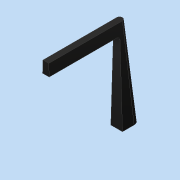
# Autodesk Inventor part: RudderStabilizingFins
Saved by Autodesk Inventor 2017 (Build 210142000, 142)
## iProperties
Created: 2016-10-10
Part Number: RudderStabilizingFins
Material: Generic
Document SubType Name: Modeling
Designer: techn
Density: 1 g/cm^3
Appearance: Glossy - Black
Author: techn
Autodesk Inventor part; units mm, degrees
ref_plane "YZ Plane" through (0, 0, 0) normal (1, 0, 0) x (0, 1, 0)
ref_plane "XY Plane" through (0, 0, 0) normal (0, 0, 1) x (1, 0, 0)
sketch "Sketch6" plane through (0, 0, 0) normal (0, 1, 0) x (-1, 0, 0)
  line L0 (0, 0) -> (6.35, 0)
  line L1 (6.35, 0) -> (6.35, -6.35)
  line L2 (6.35, -6.35) -> (0, -6.35)
  line L3 (0, -6.35) -> (0, 0)
  arc A0 (0, -6.35) -> (6.35, -6.35) centre (3.175, -6.35) ccw
  dimension "d25" = 6.35
  dimension "d26" = 6.35
  constraints: 8 end point, 2 parallel, 2 point on circle, 2 tangent, 1 centre point, 1 horizontal, 1 perpendicular
  measures "d25" distance of L1.end L2.end
  measures "d26" distance of L0.end L1.end
ref_plane "Work Plane1" through (0, 50.8, 0) normal (0, 1, 0) x (-1, 0, 0)
sketch "Sketch8" plane through (0, 50.8, 0) normal (0, 1, 0) x (-1, 0, 0)
  line L0 (4.7625, 0) -> (1.5875, 0)
  line L1 (1.5875, 0) -> (1.5875, -1.5875)
  line L2 (1.5875, -1.5875) -> (4.7625, -1.5875)
  line L3 (4.7625, -1.5875) -> (4.7625, 0)
  arc A0 (1.5875, -1.5875) -> (4.7625, -1.5875) centre (3.175, -1.5875) ccw
  point P0 (0, 0)
  dimension "d27" = 3.175
  dimension "d28" = 1.5875
  constraints: 8 end point, 2 parallel, 2 point on circle, 2 tangent, 1 centre point, 1 horizontal, 1 perpendicular, 1 point on line
  measures "d27" distance of L2.end L1.end
  measures "d28" distance of L1.end L0.end
loft "Loft1" add profiles "Sketch6", "Sketch8"
sketch "Sketch9" plane through (-6.35, 0, 0) normal (0, 0, 1) x (1, 0, 0)
  line L0 (0, 0) -> (6.35, 0) projected
  line L1 (6.35, 0) -> (4.7625, 50.8) projected
  line L2 (1.5875, 50.8) -> (4.7625, 50.8) projected
  line L3 (0, 0) -> (1.5875, 50.8) projected
  line L4 (4.7625, 50.8) -> (6.35, 0) projected
  line L5 (4.9609, 44.45) -> (1.3891, 44.45)
  line L6 (0, 0) -> (1.5875, 50.8) projected
  dimension "d34" = 6.35
  constraints: 2 end point, 2 point on line, 1 horizontal
  measures "d34" distance between parallel lines of L2 L5
extrude "Extrusion5" add sketch "Sketch9" along normal blind 38.608 contours L3 L2 L1 L5
fillet "Fillet2" radius 1.5875 1 edges at (-3.175, 44.45, 0)
sketch "Sketch12" plane through (-3.175, 0, -6.35) normal (0, -1, 0) x (1, 0, 0)
  circle A0 centre (0, 1.5875) radius 1.27
  arc A1 (-3.175, 0) -> (3.175, 0) centre (0, 0) ccw projected
  line L0 (0, -3.175) -> (0, 1.5875)
  point P0 (3.175, 6.35)
  dimension "d44" = 2.54
  dimension "d46" = 4.7625
  constraints: 2 end point, 1 centre point, 1 point on circle, 1 vertical
  measures "d44" diameter of A0
  measures "d46" distance of L0.start L0.end
extrude "Extrusion8" cut sketch "Sketch12" against normal blind 10.16
body "Solid4"
